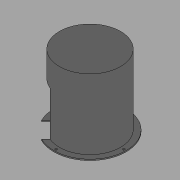
# Autodesk Inventor part: external_cover
Saved by Autodesk Inventor 2019 (Build 230136000, 136)
## iProperties
Part Number: external_cover
Material: Generic
Document SubType Name: Modeling
Designer: Javi
Appearance: Default
Author: Javi
Autodesk Inventor part; units mm, degrees
ref_plane "XZ Plane" through (0, 0, 0) normal (0, 1, 0) x (-1, 0, 0)
ref_plane "XY Plane" through (0, 0, 0) normal (0, 0, 1) x (1, 0, 0)
sketch "Sketch1" plane through (0, 0, 0) normal (0, 1, 0) x (-1, 0, 0)
  circle A0 centre (0, 0) radius 155
  dimension "d0" = 310
  constraints: 1 centre point, 1 coincident
  measures "d0" diameter of A0
extrude "Extrusion1" add sketch "Sketch1" along normal blind 305
sketch "Sketch2" plane through (0, 305, 0) normal (0, 1, 0) x (1, 0, 0)
  circle A0 centre (0, 0) radius 131
  circle A1 centre (0, 0) radius 155
  dimension "d3" = 262
  dimension "d4" = 310
  constraints: 2 centre point, 2 coincident
  measures "d3" diameter of A0
  measures "d4" diameter of A1
extrude "Extrusion2" cut sketch "Sketch2" against normal blind 300
sketch "Sketch3" plane through (0, 0, 0) normal (0, -1, 0) x (1, 0, 0)
  circle A0 centre (0, 0) radius 126
  dimension "d7" = 252
  constraints: 1 centre point, 1 coincident
  measures "d7" diameter of A0
extrude "Extrusion3" cut sketch "Sketch3" against normal blind 300
sketch "Sketch4" plane through (0, 5, 0) normal (0, 1, 0) x (1, 0, 0)
  circle A0 centre (0, 0) radius 155 projected
  line L0 (-155, 0) -> (-145, 0)
  line L1 (-155, 0) -> (-145, 0) construction
  circle A1 centre (-145, 0) radius 4.5
  circle A2 centre (0, -145) radius 4.5
  line L2 (0, -155) -> (0, -145)
  circle A3 centre (145, 0) radius 4.5
  line L3 (155, 0) -> (145, 0)
  circle A4 centre (0, 145) radius 4.5
  line L4 (0, 155) -> (0, 145)
  dimension "d10" = 10
  dimension "d12" = 9
  dimension "d15" = 360
  constraints: 10 end point, 4 centre point, 3 horizontal, 1 coincident, 1 collinear, 1 horizontal alignment, 22 other
  measures "d10" distance of L0.start L0.end
  measures "d12" diameter of A1
extrude "Extrusion4" cut sketch "Sketch4" against normal through all contours A4 | A1 | A2 | A3
ref_plane "Work Plane2" through (-109.6016, 0, 109.6016) normal (0.7071, 0, -0.7071) x (0, 1, 0)
ref_plane "Work Plane1" through (0, 0, 0) normal (0.7071, 0, -0.7071) x (0, 1, 0)
sketch "Sketch5" plane through (-109.6016, 0, 109.6016) normal (0.7071, 0, -0.7071) x (0, 1, 0)
  line L0 (195, -50) -> (0, -50)
  line L1 (0, -50) -> (0, 50)
  line L2 (0, 50) -> (195, 50)
  line L3 (195, 50) -> (195, -50)
  line L4 (0, 155) -> (0, -155) projected
  point P0 (0, 0)
  dimension "d20" = 195
  dimension "d21" = 100
  dimension "d22" = 0
  dimension "d23" = 50
  constraints: 8 end point, 2 parallel, 1 horizontal, 1 perpendicular
  measures "d20" distance of L1.end L2.end
  measures "d21" distance of L0.end L1.end
  measures "d22" distance between parallel lines of L4 L1
  measures "d23" distance from line of point (0, 0) L0
extrude "Extrusion5" cut sketch "Sketch5" along normal up to surface
body "Solid1"
